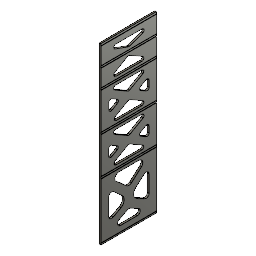
ShelfSide v17 (Autodesk Fusion 360 design; units mm, degrees)
Autodesk Fusion 360 part; units mm, degrees
(part 1 of 2)
sketch "Sketch1" plane through (0, 0, 0) normal (1, 0, 0) x (0, 0, -1)
  line L0 (-368.3, 45.5984) -> (-368.3, 1201.2984)
  line L1 (-368.3, 1201.2984) -> (0, 1201.2984)
  line L2 (0, 1201.2984) -> (0, 45.5984)
  arc A0 (857.2554, 361.5054) -> (842.4558, 407.5484) centre (842.4558, 382.1484) ccw
  arc A1 (812.2937, 264.6626) -> (813.9463, 222.6336) centre (827.3522, 244.2077) ccw
  arc A2 (735.128, 294.2271) -> (764.0591, 294.6901) centre (749.2595, 315.3331) ccw
  arc A3 (893.5104, 523.1786) -> (910.41, 535.1642) centre (897.71, 535.1642) ccw
  line L3 (910.41, 582.7318) -> (910.41, 535.1642)
  line L4 (629.9156, 458.3484) -> (854.3167, 458.3484)
  arc A4 (854.3167, 458.3484) -> (858.954, 482.8715) centre (854.3167, 471.0484) ccw
  line L5 (743.8744, 528.0081) -> (858.954, 482.8715)
  line L6 (832.5656, 544.5332) -> (893.5104, 523.1786)
  arc A5 (743.8744, 528.0081) -> (734.3905, 527.9238) centre (739.2372, 516.185) ccw
  arc A6 (910.41, 582.7318) -> (892.6921, 594.3985) centre (897.71, 582.7318) ccw
  line L7 (752.965, 591.973) -> (862.2866, 637.1096)
  line L8 (515.0777, 1201.2984) -> (515.0777, 45.5984)
  line L9 (892.6921, 594.3985) -> (831.7473, 568.1853)
  arc A7 (831.7473, 568.1853) -> (832.5656, 544.5332) centre (836.7653, 556.5187) ccw
  line L10 (972.2777, 45.5984) -> (972.2777, 1201.2984)
  arc A8 (743.481, 591.8887) -> (752.965, 591.973) centre (748.1183, 603.7118) ccw
  arc A9 (743.8475, 591.7515) -> (753.1305, 592.0427) centre (748.1183, 603.7118) ccw
  line L11 (649.4679, 407.5484) -> (842.4558, 407.5484)
  line L12 (654.1824, 552.7084) -> (583.7526, 521.2836)
  arc A10 (565.8777, 532.8814) -> (583.7526, 521.2836) centre (578.5777, 532.8814) ccw
  line L13 (582.7883, 601.0381) -> (653.2181, 576.288)
  arc A11 (642.6888, 792.4862) -> (642.0985, 816.1009) centre (637.7272, 804.1769) ccw
  arc A12 (625.0689, 482.7872) -> (629.9156, 458.3484) centre (629.9156, 471.0484) ccw
  line L14 (626.767, 966.3484) -> (860.3098, 966.3484)
  line L15 (754.5078, 830.2009) -> (907.073, 891.0521)
  line L16 (628.4015, 637.0253) -> (743.481, 591.8887)
  line L17 (625.0689, 482.7872) -> (734.3905, 527.9238)
  line L18 (565.8777, 589.0564) -> (565.8777, 532.8814)
  arc A13 (654.1824, 552.7084) -> (653.2181, 576.288) centre (649.0076, 564.3063) ccw
  arc A14 (582.7883, 601.0381) -> (565.8777, 589.0564) centre (578.5777, 589.0564) ccw
  line L19 (642.6888, 792.4862) -> (581.5349, 766.5319)
  line L20 (563.8733, 826.5959) -> (563.8733, 778.2226)
  line L21 (628.0922, 142.246) -> (712.7392, 204.6248)
  arc A15 (645.3573, 736.8447) -> (650.0623, 712.3484) centre (650.0623, 725.0484) ccw
  line L22 (572.0099, 297.7703) -> (572.0099, 216.2509)
  arc A16 (628.0922, 142.246) -> (643.1606, 96.3984) centre (643.1606, 121.7984) ccw
  arc A17 (563.8733, 778.2226) -> (581.5349, 766.5319) centre (576.5733, 778.2226) ccw
  arc A18 (672.314, 242.7586) -> (669.5625, 284.5995) centre (656.6303, 262.7382) ccw
  line L23 (610.3421, 319.6317) -> (669.5625, 284.5995)
  line L24 (580.9446, 838.5198) -> (642.0985, 816.1009)
  arc A19 (580.9446, 838.5198) -> (563.8733, 826.5959) centre (576.5733, 826.5959) ccw
  line L25 (635.3364, 361.0425) -> (735.128, 294.2271)
  arc A20 (649.4679, 407.5484) -> (635.3364, 361.0425) centre (649.4679, 382.1484) ccw
  line L26 (469.0079, 58.2984) -> (494.6168, 58.2984)
  arc A21 (633.0388, 661.5484) -> (628.4015, 637.0253) centre (633.0388, 648.8484) ccw
  line L27 (672.314, 242.7586) -> (613.0936, 196.2714)
  arc A22 (572.0099, 216.2509) -> (613.0936, 196.2714) centre (597.4099, 216.2509) ccw
  arc A23 (621.69, 990.6895) -> (626.767, 966.3484) centre (626.767, 979.0484) ccw
  arc A24 (589.8173, 915.5484) -> (585.3024, 890.9781) centre (589.8173, 902.8484) ccw
  line L28 (464.3571, 439.2984) -> (496.5151, 439.2984)
  line L29 (464.125, 693.2984) -> (492.147, 693.2984)
  line L30 (466.2488, 426.5984) -> (495.5693, 426.5984)
  line L31 (460.47, 947.2984) -> (487.2736, 947.2984)
  arc A25 (610.3421, 319.6317) -> (572.0099, 297.7703) centre (597.4099, 297.7703) ccw
  line L32 (458.0333, 934.5984) -> (487.2736, 934.5984)
  line L33 (462.9067, 680.5984) -> (493.3653, 680.5984)
  line L34 (650.0623, 712.3484) -> (837.3243, 712.3484)
  line L35 (859.147, 1169.5484) -> (625.6057, 1169.5484)
  arc A26 (862.2866, 637.1096) -> (857.4399, 661.5484) centre (857.4399, 648.8484) ccw
  arc A27 (740.9816, 205.8937) -> (712.7392, 204.6248) centre (727.8076, 184.1772) ccw
  line L36 (740.9816, 205.8937) -> (843.8091, 143.5149)
  line L37 (881.0192, 315.2571) -> (812.2937, 264.6626)
  line L38 (813.9463, 222.6336) -> (882.6719, 179.9284)
  arc A28 (837.3243, 712.3484) -> (841.8393, 736.9188) centre (837.3243, 725.0484) ccw
  arc A29 (894.9901, 770.7473) -> (912.0171, 782.6874) centre (899.3171, 782.6874) ccw
  line L39 (764.0591, 294.6901) -> (857.2554, 361.5054)
  arc A30 (745.9854, 773.3772) -> (736.7654, 773.3032) centre (741.4704, 761.5069) ccw
  arc A31 (830.6351, 96.3984) -> (843.8091, 143.5149) centre (830.6351, 121.7984) ccw
  line L40 (589.8173, 915.5484) -> (902.368, 915.5484)
  line L41 (643.1606, 96.3984) -> (830.6351, 96.3984)
  line L42 (621.69, 990.6895) -> (738.1707, 1041.4895)
  line L43 (848.2846, 787.6729) -> (894.9901, 770.7473)
  line L44 (744.6298, 1094.3609) -> (864.116, 1145.1609)
  line L45 (633.0388, 661.5484) -> (857.4399, 661.5484)
  line L46 (620.4385, 1145.2471) -> (734.4936, 1094.4471)
  line L47 (748.3034, 1041.4987) -> (865.3656, 990.6987)
  arc A32 (921.4777, 294.8022) -> (881.0192, 315.2571) centre (896.0777, 294.8022) ccw
  arc A33 (748.3034, 1041.4987) -> (738.1707, 1041.4895) centre (743.2477, 1029.8484) ccw
  line L48 (745.9854, 773.3772) -> (841.8393, 736.9188)
  line L49 (645.3573, 736.8447) -> (736.7654, 773.3032)
  arc A34 (734.4936, 1094.4471) -> (744.6298, 1094.3609) centre (739.6608, 1106.0484) ccw
  arc A35 (864.116, 1145.1609) -> (859.147, 1169.5484) centre (859.147, 1156.8484) ccw
  line L50 (456.815, 1188.5984) -> (495.802, 1188.5984)
  line L51 (461.6883, 1061.5984) -> (490.9286, 1061.5984)
  arc A36 (882.6719, 179.9284) -> (921.4777, 201.5026) centre (896.0777, 201.5026) ccw
  arc A37 (745.438, 830.0708) -> (754.723, 830.289) centre (749.8028, 841.9972) ccw
  line L52 (921.4777, 294.8022) -> (921.4777, 201.5026)
  line L53 (585.3024, 890.9781) -> (745.2878, 830.1269)
  line L54 (464.125, 1074.2984) -> (490.9286, 1074.2984)
  arc A38 (745.2878, 830.1269) -> (754.5078, 830.2009) centre (749.8028, 841.9972) ccw
  arc A39 (625.6057, 1169.5484) -> (620.4385, 1145.2471) centre (625.6057, 1156.8484) ccw
  line L55 (912.0171, 819.2253) -> (912.0171, 782.6874)
  arc A40 (907.073, 891.0521) -> (902.368, 915.5484) centre (902.368, 902.8484) ccw
  arc A41 (860.3098, 966.3484) -> (865.3656, 990.6987) centre (860.3098, 979.0484) ccw
  arc A42 (847.6946, 811.3226) -> (848.2846, 787.6729) centre (852.6116, 799.613) ccw
  line L56 (894.4001, 830.9348) -> (847.6946, 811.3226)
  arc A43 (912.0171, 819.2253) -> (894.4001, 830.9348) centre (899.3171, 819.2253) ccw
  line L57 (-250.5905, 407.5484) -> (-117.709, 407.5484)
  line L58 (-267.446, 363.1471) -> (-201.0055, 304.2097)
  line L59 (-167.2945, 304.2096) -> (-100.8535, 363.147)
  arc A44 (-250.5905, 407.5484) -> (-267.446, 363.1471) centre (-250.5905, 382.1484) ccw
  arc A45 (-100.8535, 363.147) -> (-117.709, 407.5484) centre (-117.709, 382.1484) ccw
  arc A46 (-201.0055, 304.2097) -> (-167.2945, 304.2096) centre (-184.15, 323.2111) ccw
  line L60 (-269.6734, 458.3484) -> (-98.6218, 458.3484)
  line L61 (-273.321, 661.5484) -> (-96.4416, 661.5484)
  line L62 (-279.622, 637.8218) -> (-191.1874, 587.2867)
  line L63 (-178.5858, 587.2864) -> (-90.141, 637.8215)
  line L64 (-275.974, 482.0754) -> (-190.4433, 530.9455)
  line L65 (-177.8417, 530.9452) -> (-92.3208, 482.075)
  line L66 (-298.499, 584.2184) -> (-261.3874, 563.0118)
  line L67 (-261.3874, 540.9584) -> (-298.499, 519.7517)
  line L68 (-317.5, 530.7784) -> (-317.5, 573.1917)
  line L69 (-184.1459, 534.5484) -> (-184.1459, 488.4851)
  line L70 (-69.801, 584.2184) -> (-106.9126, 563.0118)
  line L71 (-106.9126, 540.9584) -> (-69.801, 519.7517)
  line L72 (-50.8, 530.7784) -> (-50.8, 573.1917)
  arc A47 (-273.321, 661.5484) -> (-279.622, 637.8218) centre (-273.321, 648.8484) ccw
  arc A48 (-191.1874, 587.2867) -> (-178.5858, 587.2864) centre (-184.8863, 598.3133) ccw
  arc A49 (-90.141, 637.8215) -> (-96.4416, 661.5484) centre (-96.4416, 648.8484) ccw
  arc A50 (-298.499, 584.2184) -> (-317.5, 573.1917) centre (-304.8, 573.1917) ccw
  arc A51 (-317.5, 530.7784) -> (-298.499, 519.7517) centre (-304.8, 530.7784) ccw
  arc A52 (-261.3874, 540.9584) -> (-261.3874, 563.0118) centre (-267.6883, 551.9851) ccw
  arc A53 (-106.9126, 563.0118) -> (-106.9126, 540.9584) centre (-100.6117, 551.9851) ccw
  arc A54 (-50.8, 573.1917) -> (-69.801, 584.2184) centre (-63.5, 573.1917) ccw
  arc A55 (-69.801, 519.7517) -> (-50.8, 530.7784) centre (-63.5, 530.7784) ccw
  arc A56 (-177.8417, 530.9452) -> (-190.4433, 530.9455) centre (-184.1427, 519.9185) ccw
  arc A57 (-98.6218, 458.3484) -> (-92.3208, 482.075) centre (-98.6218, 471.0484) ccw
  arc A58 (-275.974, 482.0754) -> (-269.6734, 458.3484) centre (-269.6734, 471.0484) ccw
  line L73 (-297.3478, 849.3538) -> (-260.2364, 828.1472)
  arc A59 (-274.9205, 736.0697) -> (-268.6101, 712.3484) centre (-268.6101, 725.0484) ccw
  line L74 (-260.2364, 806.0938) -> (-297.3478, 784.8873)
  line L75 (-272.9377, 915.5484) -> (-98.8428, 915.5484)
  arc A60 (-260.2364, 806.0938) -> (-260.2364, 828.1472) centre (-266.5373, 817.1205) ccw
  line L76 (-279.2463, 891.8261) -> (-192.182, 841.9956)
  line L77 (-274.9205, 736.0697) -> (-189.7746, 784.821)
  arc A61 (-316.3488, 795.914) -> (-297.3478, 784.8873) centre (-303.6488, 795.914) ccw
  line L78 (-316.3488, 795.914) -> (-316.3488, 838.3271)
  arc A62 (-272.9377, 915.5484) -> (-279.2463, 891.8261) centre (-272.9377, 902.8484) ccw
  arc A63 (-92.5324, 891.8271) -> (-98.8428, 915.5484) centre (-98.8428, 902.8484) ccw
  arc A64 (-297.3478, 849.3538) -> (-316.3488, 838.3271) centre (-303.6488, 838.3271) ccw
  line L79 (-177.1557, 784.8221) -> (-91.977, 736.0708)
  line L80 (-184.147, 788.5484) -> (-184.147, 742.4851)
  line L81 (-69.8104, 846.2993) -> (-106.7924, 825.1248)
  line L82 (-106.7906, 803.0812) -> (-69.8086, 781.9148)
  arc A65 (-98.2856, 712.3484) -> (-91.977, 736.0708) centre (-98.2856, 725.0484) ccw
  arc A66 (-177.1557, 784.8221) -> (-189.7746, 784.821) centre (-183.4642, 773.7997) ccw
  arc A67 (-69.8086, 781.9148) -> (-50.8, 792.9372) centre (-63.5, 792.9372) ccw
  arc A68 (-50.8, 835.278) -> (-69.8104, 846.2993) centre (-63.5, 835.278) ccw
  line L83 (-179.5631, 841.9966) -> (-92.5324, 891.8271)
  line L84 (-50.8, 792.9372) -> (-50.8, 835.278)
  arc A69 (-106.7924, 825.1248) -> (-106.7906, 803.0812) centre (-100.482, 814.1035) ccw
  arc A70 (-192.182, 841.9956) -> (-179.5631, 841.9966) centre (-185.8735, 853.0179) ccw
  line L85 (-268.6101, 712.3484) -> (-98.2856, 712.3484)
  line L86 (-271.6979, 966.3484) -> (-98.4998, 966.3484)
  line L87 (-271.6979, 1150.4984) -> (-96.602, 1150.4984)
  line L88 (-278.238, 989.935) -> (-193.6768, 1040.735)
  line L89 (-180.8217, 1040.867) -> (-92.1848, 990.067)
  arc A71 (-180.8217, 1040.867) -> (-193.6768, 1040.735) centre (-187.1367, 1029.8484) ccw
  line L90 (0, 45.5984) -> (-368.3, 45.5984)
  line L91 (-128.1151, 96.3984) -> (-240.1849, 96.3984)
  line L92 (-249.0352, 132.3177) -> (-193.0003, 161.7159)
  line L93 (-175.2997, 161.7159) -> (-119.2648, 132.3177)
  arc A72 (-128.1151, 96.3984) -> (-119.2648, 132.3177) centre (-128.1151, 115.4484) ccw
  arc A73 (-249.0352, 132.3177) -> (-240.1849, 96.3984) centre (-240.1849, 115.4484) ccw
  arc A74 (-175.2997, 161.7159) -> (-193.0003, 161.7159) centre (-184.15, 144.8466) ccw
  line L94 (-317.5, 297.278) -> (-317.5, 185.2722)
  line L95 (-289.5997, 168.4029) -> (-237.1222, 195.9346)
  line L96 (-229.1614, 261.2792) -> (-285.8084, 311.529)
  arc A75 (-237.1222, 195.9346) -> (-229.1614, 261.2792) centre (-255.7055, 231.3558) ccw
  arc A76 (-285.8084, 311.529) -> (-317.5, 297.278) centre (-298.45, 297.278) ccw
  arc A77 (-317.5, 185.2722) -> (-289.5997, 168.4029) centre (-298.45, 185.2722) ccw
  line L97 (-184.15, 144.8466) -> (-184.15, 127.4154)
  arc A78 (-139.1386, 261.2792) -> (-131.1778, 195.9346) centre (-112.5945, 231.3558) ccw
  line L98 (-78.7003, 168.4029) -> (-131.1778, 195.9346)
  line L99 (-139.1386, 261.2792) -> (-82.4916, 311.529)
  line L100 (-50.8, 297.278) -> (-50.8, 185.2722)
  arc A79 (-78.7003, 168.4029) -> (-50.8, 185.2722) centre (-69.85, 185.2722) ccw
  arc A80 (-50.8, 297.278) -> (-82.4916, 311.529) centre (-69.85, 297.278) ccw
  line L101 (-276.0278, 1125.8593) -> (-188.4798, 1094.1093)
  line L102 (-179.8202, 1094.1093) -> (-92.2722, 1125.8593)
  arc A81 (-188.4798, 1094.1093) -> (-179.8202, 1094.1093) centre (-184.15, 1106.0484) ccw
  arc A82 (-278.238, 989.935) -> (-271.6979, 966.3484) centre (-271.6979, 979.0484) ccw
  arc A83 (-98.4998, 966.3484) -> (-92.1848, 990.067) centre (-98.4998, 979.0484) ccw
  arc A84 (-271.6979, 1150.4984) -> (-276.0278, 1125.8593) centre (-271.6979, 1137.7984) ccw
  arc A85 (-92.2722, 1125.8593) -> (-96.602, 1150.4984) centre (-96.602, 1137.7984) ccw
  point P0 (968.4898, 915.5484)
  point P1 (520.7038, 915.5484)
  point P2 (583.9405, 712.3484)
  point P3 (817.3626, 800.5791)
  point P4 (912.0171, 838.3324)
  point P5 (746.2788, 794.8984)
  point P6 (912.0171, 764.5769)
  point P7 (563.8733, 759.0362)
  point P8 (673.9106, 802.925)
  point P9 (563.8733, 844.7782)
  point P10 (746.2769, 845.6984)
  point P11 (906.4378, 712.3484)
  point P12 (921.4777, 96.3984)
  point P13 (565.8777, 96.3984)
  point P14 (515.0777, 45.5984)
  point P15 (565.8777, 661.5484)
  point P16 (743.6777, 286.8984)
  point P17 (565.8777, 458.3484)
  point P18 (746.2884, 540.8984)
  point P19 (743.6777, 217.0484)
  point P20 (910.41, 602.0192)
  point P21 (921.4777, 345.0419)
  point P22 (910.41, 517.2571)
  point P23 (778.5102, 242.5441)
  point P24 (921.4777, 407.5484)
  point P25 (921.4777, 661.5484)
  point P26 (565.8777, 606.9807)
  point P27 (565.8777, 513.308)
  point P28 (921.4777, 458.3484)
  point P29 (565.8777, 407.5484)
  point P30 (682.2269, 561.3462)
  point P31 (921.4777, 155.815)
  point P32 (805.1286, 558.5507)
  point P33 (746.2865, 591.6984)
  point P34 (921.4777, 966.3484)
  point P35 (565.8777, 966.3484)
  point P36 (746.3087, 984.25)
  point P37 (565.8777, 1169.5484)
  point P38 (921.4777, 1169.5484)
  point P39 (742.0372, 1060.45)
  point P40 (572.0099, 164.0212)
  point P41 (698.7707, 257.4348)
  point P42 (572.0099, 342.3073)
  point P43 (-317.5, 407.5484)
  point P44 (-50.7991, 407.5484)
  point P45 (-317.5, 339.6417)
  point P46 (-317.5, 458.3484)
  point P47 (-50.8, 458.3484)
  point P48 (-184.1459, 534.5484)
  point P49 (-184.1447, 585.3484)
  point P50 (-317.5, 600.9575)
  point P51 (-317.5, 516.856)
  point P52 (-243.9085, 558.9044)
  point P53 (-316.3506, 712.3484)
  point P54 (-243.2925, 812.7162)
  point P55 (-50.5291, 712.3484)
  point P56 (-316.3486, 854.5293)
  point P57 (-316.3497, 770.8864)
  point P58 (-184.1464, 839.3484)
  point P59 (-184.147, 788.5484)
  point P60 (-317.5, 966.3484)
  point P61 (-50.8, 966.3484)
  point P62 (-343.9681, 1150.4984)
  point P63 (-24.3318, 1150.4984)
  point P64 (-184.15, 1029.8484)
  point P65 (-50.8, 96.3984)
  point P66 (-317.5, 96.3984)
  point P67 (-316.3558, 338.6267)
  point P68 (-317.5, 153.7652)
  point P69 (-185.8324, 222.8433)
  point P70 (-183.5722, 1104.6817)
  dimension "d126" = 1155.7
  dimension "d127" = 457.2
  dimension "d128" = 50.8
  dimension "d130" = 50.8
  dimension "d131" = 50.8
  dimension "d132" = 50.8
  dimension "d133" = 120.65
  dimension "d134" = 228.6
  dimension "d135" = 228.6
  dimension "d136" = 120.65
  dimension "d137" = 50.8
  dimension "d138" = 50.8
  dimension "d139" = 50.8
  dimension "d140" = 50.8
  dimension "d141" = 50.8
  dimension "d142" = 50.8
  dimension "d143" = 50.8
  dimension "d144" = 50.8
  dimension "d145" = 50.8
  dimension "d146" = 25.4
  dimension "d147" = 50.8
  dimension "d148" = 50.8
  dimension "d149" = 50.8
  dimension "d150" = 50.8
  dimension "d151" = 69.85
  dimension "d152" = 50.8
  dimension "d153" = 50.8
  dimension "d154" = 50.8
  dimension "d155" = 50.8
  dimension "d156" = 50.8
  dimension "d157" = 50.8
  dimension "d158" = 50.8
  dimension "d159" = 50.8
  dimension "d160" = 50.8
  dimension "d161" = 50.8
  dimension "d162" = 12.7
  dimension "d163" = 12.7
  dimension "d164" = 12.7
  dimension "d165" = 12.7
  dimension "d166" = 12.7
  dimension "d167" = 12.7
  dimension "d168" = 69.85
  dimension "d169" = 50.8
  dimension "d170" = 50.8
  dimension "d171" = 50.8
  dimension "d172" = 50.8
  dimension "d173" = 50.8
  dimension "d174" = 50.8
  dimension "d175" = 50.8
  dimension "d176" = 50.8
  dimension "d177" = 50.8
  dimension "d178" = 12.7
  dimension "d179" = 12.7
  dimension "d180" = 12.7
  dimension "d181" = 12.7
  dimension "d182" = 12.7
  dimension "d183" = 12.7
  dimension "d184" = 50.8
  dimension "d185" = 50.8
  dimension "d186" = 12.7
  dimension "d187" = 12.7
  dimension "d188" = 12.7
  dimension "d189" = 50.8
  dimension "d190" = 50.8
  dimension "d191" = 12.7
  dimension "d192" = 368.3
  dimension "d193" = 12.7
  dimension "d194" = 19.05
  dimension "d195" = 50.8
  dimension "d196" = 241.3
  dimension "d197" = 12.7
  dimension "d198" = 19.05
  dimension "d199" = 50.8
  dimension "d200" = 241.3
  dimension "d201" = 12.7
  dimension "d202" = 50.8
  dimension "d203" = 19.05
  dimension "d204" = 114.3
  dimension "d205" = 12.7
  dimension "d206" = 114.3
  dimension "d207" = 19.05
  dimension "d208" = 12.7
  dimension "d209" = 12.7
  dimension "d210" = 12.7
  dimension "d211" = 31.75
  dimension "d212" = 31.75
  dimension "d216" = 50.8
  dimension "d218" = 19.05
  dimension "d222" = 50.8
  dimension "d223" = 50.8
  dimension "d235" = 25.4
  dimension "d236" = 25.4
  dimension "d237" = 25.4
  dimension "d273" = 368.3
  dimension "d282" = 117.7095
  dimension "d283" = 117.709
  dimension "d284" = 184.15
  dimension "d287" = 50.8
  dimension "d288" = 50.8
  dimension "d289" = 50.8
  dimension "d290" = 203.2
  dimension "d291" = 50.8
  dimension "d292" = 76.2
  dimension "d293" = 50.8
  dimension "d294" = 50.8
  dimension "d295" = 50.8
  dimension "d296" = 50.8
  dimension "d297" = 50.8
  dimension "d298" = 50.8
  dimension "d299" = 12.7
  dimension "d300" = 12.7
  dimension "d301" = 12.7
  dimension "d302" = 12.7
  dimension "d303" = 12.7
  dimension "d304" = 12.7
  dimension "d305" = 12.7
  dimension "d306" = 12.7
  dimension "d307" = 12.7
  dimension "d308" = 12.7
  dimension "d309" = 12.7
  dimension "d310" = 12.7
  dimension "d312" = 203.2
  dimension "d313" = 50.8
  dimension "d314" = 76.2
  dimension "d315" = 50.8
  dimension "d316" = 50.8
  dimension "d319" = 50.8
  dimension "d320" = 50.8
  dimension "d321" = 12.7
  dimension "d322" = 12.7
  dimension "d323" = 12.7
  dimension "d324" = 12.7
  dimension "d325" = 12.7
  dimension "d326" = 12.7
  dimension "d327" = 12.7
  dimension "d328" = 12.7
  dimension "d329" = 12.7
  dimension "d330" = 12.7
  dimension "d331" = 12.7
  dimension "d332" = 12.7
  dimension "d333" = 50.8
  dimension "d334" = 50.8
  dimension "d335" = 50.8
  dimension "d337" = 50.8
  dimension "d338" = 50.8
  dimension "d339" = 50.8
  dimension "d340" = 50.8
  dimension "d344" = 12.7
  dimension "d345" = 31.75
  dimension "d352" = 12.7
  dimension "d353" = 1155.7
  dimension "d354" = 50.8
  dimension "d355" = 50.8
  dimension "d356" = 19.05
  dimension "d357" = 19.05
  dimension "d358" = 19.05
  dimension "d362" = 50.8
  dimension "d363" = 50.8
  dimension "d364" = 50.8
  dimension "d365" = 50.8
  dimension "d366" = 50.8
  dimension "d367" = 40
  dimension "d368" = 19.05
  dimension "d369" = 19.05
  dimension "d370" = 50.8
  dimension "d371" = 12.7
  dimension "d372" = 31.75
  dimension "d373" = 12.7
  dimension "d374" = 12.7
  dimension "d375" = 12.7
  dimension "d376" = 12.7
  dimension "d379" = 50.8
  dimension "d380" = 173.1981
  dimension "d382" = 184.15
  dimension "d383" = 96.6021
  dimension "d384" = 96.6021
  dimension "d385" = 96.602
  measures "d126" distance of P14 L8.start
  measures "d127" distance of P14 L10.start
  measures "d128" distance of P13 L8
  measures "d130" distance of P12 L10
  measures "d131" distance of P29 L8
  measures "d132" distance of P24 L10
  measures "d133" distance of P16 L11
  measures "d134" distance of P16 L8
  measures "d135" distance of P19 L8
  measures "d136" distance of P19 L41
  measures "d137" distance of L10 L52
  measures "d138" distance of P21 L39
  measures "d139" distance of P31 L36
  measures "d140" distance of P23 L36
  measures "d141" distance of P23 L39
  measures "d142" distance of P40 L21
  measures "d143" distance of P42 L25
  measures "d144" distance of P41 L25
  measures "d145" distance of P41 L21
  measures "d146" radius of A25
  measures "d147" distance of P17 L8
  measures "d148" distance of P28 L10
  measures "d149" distance of P15 L8
  measures "d150" distance of P25 L10
  measures "d151" distance of P33 L45
  measures "d152" distance of P18 P33
  measures "d153" distance of P20 L7
  measures "d154" distance of P22 L5
  measures "d155" distance of P32 L7
  measures "d156" distance of P32 L5
  measures "d157" distance of L8 L18
  measures "d158" distance of P26 L16
  measures "d159" distance of P27 L17
  measures "d160" distance of P30 L16
  measures "d161" distance of P30 L17
  measures "d162" radius of A9
  measures "d163" radius of A8
  measures "d164" radius of A21
  measures "d165" radius of A7
  measures "d166" radius of A14
  measures "d167" radius of A5
  measures "d168" distance of P10 L40
  measures "d169" distance of P5 P10
  measures "d170" distance of P4 L15
  measures "d171" distance of P6 L48
  measures "d172" distance of P3 L15
  measures "d173" distance of P3 L48
  measures "d174" distance of P9 L53
  measures "d175" distance of P7 L49
  measures "d176" distance of P8 L53
  measures "d177" distance of P8 L49
  measures "d178" radius of A37
  measures "d179" radius of A38
  measures "d180" radius of A24
  measures "d181" radius of A42
  measures "d182" radius of A19
  measures "d183" radius of A30
  measures "d184" distance of P35 L8
  measures "d185" distance of P34 L10
  measures "d186" radius of A33
  measures "d187" radius of A41
  measures "d188" radius of A23
  measures "d189" distance of P37 L8
  measures "d190" distance of P38 L10
  measures "d191" distance of P14 L26
  measures "d192" distance of L26 L30
  measures "d193" distance of L28 L30
  measures "d194" distance of L30.end L11
  measures "d195" distance of L4 L11
  measures "d196" distance of L28 L33
  measures "d197" distance of L29 L33
  measures "d198" distance of L33 L45
  measures "d199" distance of L34 L45
  measures "d200" distance of L29 L32
  measures "d201" distance of L31 L32
  measures "d202" distance of L14 L40
  measures "d203" distance of L32 L40
  measures "d204" distance of L31 L51
  measures "d205" distance of L51 L54
  measures "d206" distance of L50 L54
  measures "d207" distance of L35 L50
  measures "d208" radius of A39
  measures "d209" radius of A35
  measures "d210" radius of A34
  measures "d211" distance of A33.centre L51
  measures "d212" distance of A34.centre L54
  measures "d216" distance of L0 P43
  measures "d218" distance of L30 L57
  measures "d222" distance of L58 P45
  measures "d223" distance of L0 P45
  measures "d235" radius of A44
  measures "d236" radius of A45
  measures "d237" radius of A46
  measures "d273" distance of L0.end L1.end
  measures "d282" distance of L0 A44.centre
  measures "d283" distance of L2 A45.centre
  measures "d284" distance of L2 A46.centre
  measures "d287" distance of L0 P46
  measures "d288" distance of L2 P47
  measures "d289" distance of L57 L60
  measures "d290" distance of L60 L61
  measures "d291" distance of P48 P49
  measures "d292" distance of L60 P48
  measures "d293" distance of L62 P50
  measures "d294" distance of L64 P51
  measures "d295" distance of L0 P50
  measures "d296" distance of L0 P51
  measures "d297" distance of L62 P52
  measures "d298" distance of L64 P52
  measures "d299" radius of A47
  measures "d300" radius of A48
  measures "d301" radius of A49
  measures "d302" radius of A50
  measures "d303" radius of A51
  measures "d304" radius of A52
  measures "d305" radius of A53
  measures "d306" radius of A54
  measures "d307" radius of A55
  measures "d308" radius of A56
  measures "d309" radius of A57
  measures "d310" radius of A58
  measures "d312" distance of L75 L85
  measures "d313" distance of P58 P59
  measures "d314" distance of P59 L85
  measures "d315" distance of P56 L76
  measures "d316" distance of P57 L77
  measures "d319" distance of P54 L76
  measures "d320" distance of P54 L77
  measures "d321" radius of A62
  measures "d322" radius of A70
  measures "d323" radius of A63
  measures "d324" radius of A64
  measures "d325" radius of A61
  measures "d326" radius of A60
  measures "d327" radius of A69
  measures "d328" radius of A68
  measures "d329" radius of A67
  measures "d330" radius of A66
  measures "d331" radius of A65
  measures "d332" radius of A59
  measures "d333" distance of L61 L85
  measures "d334" distance of L79 L82
  measures "d335" distance of L81 L83
  measures "d337" distance of L2 A68.start
  measures "d338" distance of L2 A67.end
  measures "d339" distance of L0 P60
  measures "d340" distance of L2 P61
  measures "d344" radius of A71
  measures "d345" distance of L51 A71.centre
  measures "d352" distance of L26 L90
  measures "d353" distance of L1 L90
  measures "d354" distance of L0 P66
  measures "d355" distance of L2 P65
  measures "d356" radius of A72
  measures "d357" radius of A73
  measures "d358" radius of A74
  measures "d362" distance of L0 P68
  measures "d363" distance of L92 P68
  measures "d364" distance of L58 P67
  measures "d365" distance of L58 P69
  measures "d366" distance of L92 P69
  measures "d367" radius of A75
  measures "d368" radius of A76
  measures "d369" radius of A77
  measures "d370" distance of L1 L87
  measures "d371" radius of A81
  measures "d372" distance of L54 A81.centre
  measures "d373" radius of A82
  measures "d374" radius of A83
  measures "d375" radius of A84
  measures "d376" radius of A85
  measures "d379" distance of L75 L86
  measures "d380" distance of A82.centre A83.centre
  measures "d382" distance of L2 A81.centre
  measures "d383" distance of L0 A82.centre
  measures "d384" distance of L0 A84.centre
  measures "d385" distance of L2 A85.centre
extrude "Extrude2" add sketch "Sketch1" along normal blind 12.7 contours L0 L1 L2 L90
sketch "Sketch2" plane through (12.7, 0, 0) normal (1, 0, 0) x (0, 0, -1)
  arc A0 (-271.6979, 1150.4984) -> (-276.0278, 1125.8593) centre (-271.6979, 1137.7984) ccw
  line L0 (-271.6979, 1150.4984) -> (-96.602, 1150.4984)
  arc A1 (-92.2722, 1125.8593) -> (-96.602, 1150.4984) centre (-96.602, 1137.7984) ccw
  line L1 (-92.2722, 1125.8593) -> (-179.8202, 1094.1093)
  arc A2 (-188.4798, 1094.1093) -> (-179.8202, 1094.1093) centre (-184.15, 1106.0484) ccw
  line L2 (-188.4798, 1094.1093) -> (-276.0278, 1125.8593)
  arc A3 (-128.1151, 96.3984) -> (-119.2648, 132.3177) centre (-128.1151, 115.4484) ccw
  line L3 (-128.1151, 96.3984) -> (-240.1849, 96.3984)
  arc A4 (-249.0352, 132.3177) -> (-240.1849, 96.3984) centre (-240.1849, 115.4484) ccw
  line L4 (-249.0352, 132.3177) -> (-193.0003, 161.7159)
  arc A5 (-175.2997, 161.7159) -> (-193.0003, 161.7159) centre (-184.15, 144.8466) ccw
  line L5 (-175.2997, 161.7159) -> (-119.2648, 132.3177)
  arc A6 (-78.7003, 168.4029) -> (-50.8, 185.2722) centre (-69.85, 185.2722) ccw
  line L6 (-78.7003, 168.4029) -> (-131.1778, 195.9346)
  arc A7 (-139.1386, 261.2792) -> (-131.1778, 195.9346) centre (-112.5945, 231.3558) ccw
  line L7 (-139.1386, 261.2792) -> (-82.4916, 311.529)
  arc A8 (-50.8, 297.278) -> (-82.4916, 311.529) centre (-69.85, 297.278) ccw
  line L8 (-50.8, 297.278) -> (-50.8, 185.2722)
  arc A9 (-278.238, 989.935) -> (-271.6979, 966.3484) centre (-271.6979, 979.0484) ccw
  line L9 (-278.238, 989.935) -> (-193.6768, 1040.735)
  arc A10 (-180.8217, 1040.867) -> (-193.6768, 1040.735) centre (-187.1367, 1029.8484) ccw
  line L10 (-180.8217, 1040.867) -> (-92.1848, 990.067)
  arc A11 (-98.4998, 966.3484) -> (-92.1848, 990.067) centre (-98.4998, 979.0484) ccw
  line L11 (-98.4998, 966.3484) -> (-271.6979, 966.3484)
  arc A12 (-317.5, 185.2722) -> (-289.5997, 168.4029) centre (-298.45, 185.2722) ccw
  line L12 (-317.5, 185.2722) -> (-317.5, 297.278)
  arc A13 (-285.8084, 311.529) -> (-317.5, 297.278) centre (-298.45, 297.278) ccw
  line L13 (-285.8084, 311.529) -> (-229.1614, 261.2792)
  arc A14 (-237.1222, 195.9346) -> (-229.1614, 261.2792) centre (-255.7055, 231.3558) ccw
  line L14 (-237.1222, 195.9346) -> (-289.5997, 168.4029)
  arc A15 (-260.2364, 806.0938) -> (-260.2364, 828.1472) centre (-266.5373, 817.1205) ccw
  line L15 (-260.2364, 806.0938) -> (-297.3478, 784.8873)
  arc A16 (-316.3488, 795.914) -> (-297.3478, 784.8873) centre (-303.6488, 795.914) ccw
  line L16 (-316.3488, 795.914) -> (-316.3488, 838.3271)
  arc A17 (-297.3478, 849.3538) -> (-316.3488, 838.3271) centre (-303.6488, 838.3271) ccw
  line L17 (-297.3478, 849.3538) -> (-260.2364, 828.1472)
  arc A18 (-274.9205, 736.0697) -> (-268.6101, 712.3484) centre (-268.6101, 725.0484) ccw
  line L18 (-274.9205, 736.0697) -> (-189.7746, 784.821)
  arc A19 (-177.1557, 784.8221) -> (-189.7746, 784.821) centre (-183.4642, 773.7997) ccw
  line L19 (-177.1557, 784.8221) -> (-91.977, 736.0708)
  arc A20 (-98.2856, 712.3484) -> (-91.977, 736.0708) centre (-98.2856, 725.0484) ccw
  line L20 (-98.2856, 712.3484) -> (-268.6101, 712.3484)
  arc A21 (-106.7924, 825.1248) -> (-106.7906, 803.0812) centre (-100.482, 814.1035) ccw
  line L21 (-106.7924, 825.1248) -> (-69.8104, 846.2993)
  arc A22 (-50.8, 835.278) -> (-69.8104, 846.2993) centre (-63.5, 835.278) ccw
  line L22 (-50.8, 835.278) -> (-50.8, 792.9372)
  arc A23 (-69.8086, 781.9148) -> (-50.8, 792.9372) centre (-63.5, 792.9372) ccw
  line L23 (-69.8086, 781.9148) -> (-106.7906, 803.0812)
  arc A24 (-273.321, 661.5484) -> (-279.622, 637.8218) centre (-273.321, 648.8484) ccw
  line L24 (-273.321, 661.5484) -> (-96.4416, 661.5484)
  arc A25 (-90.141, 637.8215) -> (-96.4416, 661.5484) centre (-96.4416, 648.8484) ccw
  line L25 (-90.141, 637.8215) -> (-178.5858, 587.2864)
  arc A26 (-191.1874, 587.2867) -> (-178.5858, 587.2864) centre (-184.8863, 598.3133) ccw
  line L26 (-191.1874, 587.2867) -> (-279.622, 637.8218)
  arc A27 (-69.801, 519.7517) -> (-50.8, 530.7784) centre (-63.5, 530.7784) ccw
  line L27 (-69.801, 519.7517) -> (-106.9126, 540.9584)
  arc A28 (-106.9126, 563.0118) -> (-106.9126, 540.9584) centre (-100.6117, 551.9851) ccw
  line L28 (-106.9126, 563.0118) -> (-69.801, 584.2184)
  arc A29 (-50.8, 573.1917) -> (-69.801, 584.2184) centre (-63.5, 573.1917) ccw
  line L29 (-50.8, 573.1917) -> (-50.8, 530.7784)
  arc A30 (-177.8417, 530.9452) -> (-190.4433, 530.9455) centre (-184.1427, 519.9185) ccw
  line L30 (-177.8417, 530.9452) -> (-92.3208, 482.075)
  arc A31 (-98.6218, 458.3484) -> (-92.3208, 482.075) centre (-98.6218, 471.0484) ccw
  line L31 (-98.6218, 458.3484) -> (-269.6734, 458.3484)
  arc A32 (-275.974, 482.0754) -> (-269.6734, 458.3484) centre (-269.6734, 471.0484) ccw
  line L32 (-275.974, 482.0754) -> (-190.4433, 530.9455)
  arc A33 (-250.5905, 407.5484) -> (-267.446, 363.1471) centre (-250.5905, 382.1484) ccw
  line L33 (-250.5905, 407.5484) -> (-117.709, 407.5484)
  arc A34 (-100.8535, 363.147) -> (-117.709, 407.5484) centre (-117.709, 382.1484) ccw
  line L34 (-100.8535, 363.147) -> (-167.2945, 304.2096)
  arc A35 (-201.0055, 304.2097) -> (-167.2945, 304.2096) centre (-184.15, 323.2111) ccw
  line L35 (-201.0055, 304.2097) -> (-267.446, 363.1471)
  arc A36 (-317.5, 530.7784) -> (-298.499, 519.7517) centre (-304.8, 530.7784) ccw
  line L36 (-317.5, 530.7784) -> (-317.5, 573.1917)
  arc A37 (-298.499, 584.2184) -> (-317.5, 573.1917) centre (-304.8, 573.1917) ccw
  line L37 (-298.499, 584.2184) -> (-261.3874, 563.0118)
  arc A38 (-261.3874, 540.9584) -> (-261.3874, 563.0118) centre (-267.6883, 551.9851) ccw
  line L38 (-261.3874, 540.9584) -> (-298.499, 519.7517)
  arc A39 (-272.9377, 915.5484) -> (-279.2463, 891.8261) centre (-272.9377, 902.8484) ccw
  line L39 (-272.9377, 915.5484) -> (-98.8428, 915.5484)
  arc A40 (-92.5324, 891.8271) -> (-98.8428, 915.5484) centre (-98.8428, 902.8484) ccw
  line L40 (-92.5324, 891.8271) -> (-179.5631, 841.9966)
  arc A41 (-192.182, 841.9956) -> (-179.5631, 841.9966) centre (-185.8735, 853.0179) ccw
  line L41 (-192.182, 841.9956) -> (-279.2463, 891.8261)
  line L42 (0, 45.5984) -> (0, 1201.2984)
  line L43 (0, 1201.2984) -> (-368.3, 1201.2984)
  line L44 (-368.3, 1201.2984) -> (-368.3, 45.5984)
  line L45 (-368.3, 45.5984) -> (0, 45.5984)
  line L46 (0, 1074.2984) -> (-368.3, 1074.2984)
  line L47 (-368.3, 1074.2984) -> (-368.3, 1061.2984)
  line L48 (-368.3, 1061.2984) -> (0, 1061.2984)
  line L49 (0, 1061.2984) -> (0, 1074.2984)
  line L50 (-368.3, 1201.2984) -> (0, 1201.2984)
  line L51 (-368.3, 45.5984) -> (-368.3, 1201.2984)
  line L52 (0, 1201.2984) -> (0, 45.5984)
  line L53 (-388.3577, 947.2984) -> (39.0964, 947.2984)
  line L54 (39.0964, 947.2984) -> (39.0964, 934.2984)
  line L55 (39.0964, 934.2984) -> (-388.3577, 934.2984)
  line L56 (-388.3577, 934.2984) -> (-388.3577, 947.2984)
  line L57 (-368.3, 693.2984) -> (0, 693.2984)
  line L58 (0, 693.2984) -> (0, 680.2984)
  line L59 (0, 680.2984) -> (-368.3, 680.2984)
  line L60 (-368.3, 680.2984) -> (-368.3, 693.2984)
  line L61 (-368.3, 439.2984) -> (0, 439.2984)
  line L62 (0, 439.2984) -> (0, 426.2984)
  line L63 (0, 426.2984) -> (-368.3, 426.2984)
  line L64 (-368.3, 426.2984) -> (-368.3, 439.2984)
  line L65 (-368.3, 58.2984) -> (21.1472, 58.2984)
  line L66 (21.1472, 58.2984) -> (21.1472, 23.3895)
  line L67 (21.1472, 23.3895) -> (-368.3, 23.3895)
  line L68 (-368.3, 23.3895) -> (-368.3, 58.2984)
  line L69 (-368.3, 1201.2984) -> (0, 1201.2984)
  line L70 (0, 1201.2984) -> (0, 1188.2984)
  line L71 (0, 1188.2984) -> (-368.3, 1188.2984)
  line L72 (-368.3, 1188.2984) -> (-368.3, 1201.2984)
  dimension "d386" = 127
  dimension "d387" = 13
  dimension "d390" = 13
  dimension "d392" = 13
  dimension "d394" = 13
  dimension "d395" = 127
  dimension "d396" = 254
  dimension "d397" = 254
  dimension "d398" = 381
  dimension "d399" = 13
  measures "d386" distance of L46 L50
  measures "d387" distance of L46.start L48.end
  measures "d390" distance of L53.end L54.end
  measures "d392" distance of L57.end L58.end
  measures "d394" distance of L61.end L62.end
  measures "d395" distance of L46 L53
  measures "d396" distance of L53 L57
  measures "d397" distance of L57 L61
  measures "d398" distance of L61 L65
  measures "d399" distance of L43.end L71.end
extrude "Extrude4" cut sketch "Sketch2" against normal blind 2 contours L42 L44 L51 L52 L61 L62 L63 L64 | L42 L44 L45 L51 L52 L65 L68 | L42 L44 L51 L52 L57 L58 L59 L60 | L42 L44 L51 L52 L53 L55 | L42 L44 L46 L47 L48 L49 L51 L52 | L42 L43 L44 L50 L51 L52 L69 L70 L71 L72
sketch "Sketch3" plane through (0, 693.2984, 0) normal (0, -1, 0) x (1, 0, 0)
  line L0 (12.7, 0) -> (12.7, 368.3)
  line L1 (12.7, 368.3) -> (10.7, 368.3)
  line L2 (10.7, 368.3) -> (10.7, 0)
  line L3 (10.7, 0) -> (12.7, 0)
sketch "Sketch4" plane through (12.7, 0, 0) normal (1, 0, 0) x (0, 0, -1)
  arc A0 (-271.6979, 1150.4984) -> (-276.0278, 1125.8593) centre (-271.6979, 1137.7984) ccw
  line L0 (-271.6979, 1150.4984) -> (-96.602, 1150.4984)
  arc A1 (-92.2722, 1125.8593) -> (-96.602, 1150.4984) centre (-96.602, 1137.7984) ccw
  line L1 (-92.2722, 1125.8593) -> (-179.8202, 1094.1093)
  arc A2 (-188.4798, 1094.1093) -> (-179.8202, 1094.1093) centre (-184.15, 1106.0484) ccw
  line L2 (-188.4798, 1094.1093) -> (-276.0278, 1125.8593)
  line L3 (-368.3, 1074.2984) -> (0, 1074.2984)
  line L4 (0, 1074.2984) -> (0, 1188.2984)
  line L5 (0, 1188.2984) -> (-368.3, 1188.2984)
  line L6 (-368.3, 1188.2984) -> (-368.3, 1074.2984)
sketch "Sketch5" plane through (0, 0, 317.5) normal (0, 0, -1) x (-1, 0, 0)
  line L0 (0, 185.2722) -> (0, 297.278)
  line L1 (0, 297.278) -> (-12.7, 297.278)
  line L2 (-12.7, 297.278) -> (-12.7, 185.2722)
  line L3 (-12.7, 185.2722) -> (0, 185.2722)
sketch "Sketch6" plane through (12.7, 1131.2984, 184.15) normal (1, 0, 0) x (0, 0, -1)